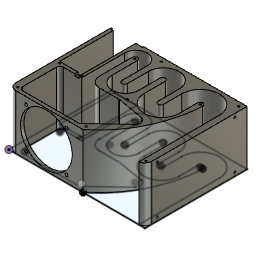
hifi_Back_horn_2_v2 v2 (Autodesk Fusion 360 design; units mm, degrees)
Autodesk Fusion 360 part; units mm, degrees
other "Fonction de maillage de base1"
sketch "Sketch1" plane through (0, 0, 0) normal (0, 0, 1) x (1, 0, 0)
  line L0 (0, 0) -> (200, 0)
  line L1 (200, 0) -> (200, 150)
  line L2 (200, 150) -> (0, 150)
  line L3 (0, 150) -> (0, 0)
  line L4 (42, 65) -> (42, 128)
  line L5 (53, 128) -> (53, 80)
  line L6 (61, 128) -> (61, 91)
  line L7 (75, 128) -> (75, 91)
  line L8 (83, 122) -> (83, 91)
  line L9 (100, 122) -> (100, 91)
  line L10 (108, 122) -> (108, 91)
  line L11 (128, 122) -> (128, 91)
  line L12 (136, 118) -> (136, 91)
  line L13 (159, 118) -> (159, 91)
  line L14 (191, 118) -> (191, 0)
  line L15 (136.3, 58.3) -> (97.4773, 65.0059)
  line L16 (140.5, 44.6) -> (99.9689, 6.2717)
  line L17 (96.6373, 5) -> (15, 5)
  line L18 (10, 10) -> (10, 60)
  line L19 (15, 65) -> (42, 65)
  line L20 (68, 65) -> (96.5085, 65)
  arc A0 (15, 65) -> (10, 60) centre (15, 60) ccw
  arc A1 (10, 10) -> (15, 5) centre (15, 10) ccw
  arc A2 (96.6373, 5) -> (99.9689, 6.2717) centre (96.6373, 10) ccw
  arc A3 (140.5, 44.6) -> (136.3, 58.3) centre (134.9332, 50.3872) ccw
  arc A4 (53, 80) -> (68, 65) centre (68, 80) ccw
  arc A5 (75, 91) -> (83, 91) centre (79, 91) ccw
  arc A6 (61, 91) -> (100, 91) centre (80.5, 91) ccw
  arc A7 (128, 122) -> (83, 122) centre (105.5, 122) ccw
  arc A8 (128, 91) -> (136, 91) centre (132, 91) ccw
  arc A9 (108, 91) -> (159, 91) centre (133.5, 91) ccw
  arc A10 (108, 122) -> (100, 122) centre (104, 122) ccw
  arc A11 (75, 128) -> (42, 128) centre (58.5, 128) ccw
  arc A12 (61, 128) -> (53, 128) centre (57, 128) ccw
  arc A13 (191, 118) -> (136, 118) centre (163.5, 118) ccw
  line L21 (96.5085, 65) -> (97.4773, 65.0059)
  spline S0 degree 5 poles (167, 118) (167, 115.0317) (166.6746, 108.5042) (165.211, 96.9417) (161.2879, 78.5371) (152.1463, 52.6808) (139.7381, 31.2801) (126.2481, 15.4712) (115.1076, 5.1248) (109, 0) knots 0 0 0 0 0 0 0.2 0.4 0.6 0.8 1 1 1 1 1 1
  line L22 (123.9379, 12.5344) -> (94.0621, -12.5344)
  line L23 (167, 125.2) -> (167, 110.8)
  arc A14 (167, 118) -> (159, 118) centre (163, 118) ccw
  line L24 (5, 150) -> (38, 150)
  line L25 (38, 150) -> (38, 69.5)
  line L26 (38, 69.5) -> (5, 69.5)
  line L27 (5, 69.5) -> (5, 150)
  line L28 (38, 69.5) -> (35, 69.5)
  line L29 (35, 69.5) -> (35, 65)
  line L30 (35, 65) -> (38, 65)
  line L31 (38, 65) -> (38, 69.5)
  point P0 (167, 118)
  dimension "d1" = 200
  dimension "d2" = 150
  dimension "d3" = 10
  dimension "d4" = 5
  dimension "d5" = 60
  dimension "d6" = 60
  dimension "d7" = 9
  dimension "d8" = 42
  dimension "d9" = 11
  dimension "d10" = 8
  dimension "d11" = 14
  dimension "d12" = 8
  dimension "d13" = 17
  dimension "d14" = 8
  dimension "d15" = 20
  dimension "d16" = 8
  dimension "d17" = 23
  dimension "d18" = 8
  dimension "d19" = 28
  dimension "d20" = 31
  dimension "d21" = 44.6
  dimension "d22" = 59.5
  dimension "d23" = 46.6
  dimension "d24" = 58.3
  dimension "d25" = 63.7
  dimension "d26" = 9.8
  dimension "d27" = 63
  dimension "d28" = 27
  dimension "d29" = 48
  dimension "d30" = 15
  dimension "d31" = 5
  dimension "d32" = 5
  dimension "d33" = 5
  dimension "d34" = 91
  dimension "d35" = 140
  dimension "d36" = 39
  dimension "d37" = 14.4
  dimension "d54" = 5
  dimension "d55" = 33
  dimension "d56" = 4.5
  dimension "d57" = 3
  constraint horizontal L0
  constraint vertical L1
  constraint horizontal L2
  constraint vertical L3
  constraint coincident L0.start L3.end
  constraint vertical L4
  constraint vertical L5
  constraint vertical L6
  constraint vertical L7
  constraint vertical L8
  constraint vertical L9
  constraint vertical L10
  constraint vertical L11
  constraint vertical L12
  constraint vertical L13
  constraint coincident L0 L14.end
  constraint perpendicular L0 L14
  constraint parallel L0 L17
  constraint perpendicular L17 L18
  constraint horizontal L20
  constraint horizontal L19
  constraint horizontal L13.start P0
  constraint horizontal L8.start L9.start
  constraint horizontal L9.start L10.start
  constraint horizontal L10.start L11.start
  constraint horizontal L7.end L8.end
  constraint horizontal L6.end L8.end
  constraint horizontal L6.end L10.end
  constraint horizontal L10.end L11.end
  constraint horizontal L11.end L12.end
  constraint horizontal L12.end L13.end
  constraint horizontal L8.end L9.end
  constraint tangent L18 A0
  constraint tangent L18 A1
  constraint tangent L17 A2
  constraint tangent L15 A3
  constraint tangent L20 A4
  constraint tangent L7 A5
  constraint tangent L6 A6
  constraint tangent L8 A7
  constraint tangent L11 A8
  constraint tangent L10 A9
  constraint tangent L9 A10
  constraint horizontal L5.start L6.start
  constraint horizontal L6.start L7.start
  constraint horizontal L4.end L5.start
  constraint tangent L4 A11
  constraint tangent L5 A12
  constraint horizontal L12.start L13.start
  constraint horizontal L14.start P0
  constraint tangent L12 A13
  constraint tangent L17 A1
  constraint tangent L19 A0
  constraint coincident P0 S0.start
  constraint coincident L0 S0.end
  constraint midpoint S0.end L22
  constraint midpoint P0 L23
  constraint vertical L23
  constraint tangent L13 A14
  constraint horizontal L24
  constraint vertical L25
  constraint horizontal L26
  constraint vertical L27
  constraint coincident L2 L24.start
  constraint horizontal L28
  constraint vertical L29
  constraint horizontal L30
  constraint vertical L31
  constraint coincident L19 L29.end
  measures "d1" distance of L0.start L0.end
  measures "d2" distance of L0.start L2.end
  measures "d3" distance of L3 L18
  measures "d4" distance of L0 L17
  measures "d5" distance of L17 L19
  measures "d6" distance of L17 L20
  measures "d7" distance of L1 L14
  measures "d8" distance of L3 L4
  measures "d9" distance of L4 L5
  measures "d10" distance of L5 L6
  measures "d11" distance of L6 L7
  measures "d12" distance of L7 L8
  measures "d13" distance of L8 L9
  measures "d14" distance of L9 L10
  measures "d15" distance of L10 L11
  measures "d16" distance of L11 L12
  measures "d17" distance of L12 L13
  measures "d18" distance of L13.start P0
  measures "d19" distance of L2 L9.start
  measures "d20" distance of L9.start L9.end
  measures "d21" distance of L0 L16.start
  measures "d22" distance of L1 L16.start
  measures "d23" angle of L1 L16
  measures "d24" distance of L0 L15.start
  measures "d25" distance of L1 L15.start
  measures "d26" angle of L15 L20
  measures "d27" distance of L4.start L4.end
  measures "d28" distance of L12.start L12.end
  measures "d29" distance of L5.start L5.end
  measures "d30" distance of L5 L20.start
  measures "d31" distance of L17 L18.start
  measures "d32" radius of A0
  measures "d33" radius of A2
  measures "d34" distance of L0.end S0.end
  measures "d35" angle of L0 L22
  measures "d36" distance of L22.start L22.end
  measures "d37" distance of L23.start L23.end
  measures "d54" distance of L3 L27
  measures "d55" distance of L25.end L26.end
  measures "d56" distance of L19 L26
  measures "d57" distance of L29 L31
extrude "Extrude1" add sketch "Sketch1" along normal blind 80 contours L0 L2 L3 L5 L6 L9 L10 L13 L15 L16 L17 L18 L19 L20 A0 A1 A2 A3 A4 A6 A9 A10 A12 L21 S0 A14 L26 L27 L29 | L0 L1 L2 L4 L7 L8 L11 L12 L14 L19 A5 A7 A8 A11 A13 L25 L31 | L19 L26 L28 L29 L30 L31
sketch "Sketch2" plane through (0, 0, 0) normal (0, 1, 0) x (1, 0, 0)
  circle A0 centre (55, -40) radius 38
  line L0 (42, 0) -> (75, 0)
  line L1 (55, -40) -> (55, 0) construction
  circle A1 centre (25.3015, -10.3015) radius 2.15
  line L2 (25.3015, -10.3015) -> (55, -40) construction
  circle A2 centre (25.3015, -69.6985) radius 2.15
  circle A3 centre (84.6985, -69.6985) radius 2.15
  circle A4 centre (84.6985, -10.3015) radius 2.15
  dimension "d40" = 76
  dimension "d41" = 40
  dimension "d42" = 55
  dimension "d43" = 4.3
  dimension "d44" = 42
  dimension "d45" = 45
  dimension "d47" = 360
  constraint coincident A0.centre L1.start
  constraint coincident L0 L1.end
  constraint vertical L1
  constraint coincident A1.centre L2.start
  measures "d40" diameter of A0
  measures "d41" distance of A0.centre L1.end
  measures "d42" distance of origin L1
  measures "d43" diameter of A1
  measures "d44" distance of A0.centre A1.centre
  measures "d45" angle of L1 L2
extrude "Extrude2" cut sketch "Sketch2" along normal up to surface (5 mm away)
fillet "Fillet1" radius 10 1 edges at (200, 0, 40)
fillet "Fillet2" radius 10 1 edges at (0, 0, 40)
extrude "Extrude3" cut sketch "Sketch1" against normal blind 3 from surface at 80 contours L19 L26 L28 L29 L30 L31
sketch "Sketch3" plane through (200, 0, 0) normal (1, 0, 0) x (0, 1, 0)
  line L0 (9.9499, 80) -> (9.9499, 0)
  line L1 (9.9499, 0) -> (150, 0)
  line L2 (150, 0) -> (150, 80)
  line L3 (150, 80) -> (9.9499, 80)
  circle A0 centre (18, 75) radius 1.5
  circle A1 centre (18, 5) radius 1.5
  circle A2 centre (132, 5) radius 1.5
  circle A3 centre (132, 75) radius 1.5
  line L4 (0, 0) -> (150, 0)
  line L5 (0, 0) -> (0, 80)
  dimension "d61" = 3
  dimension "d62" = 3
  dimension "d63" = 3
  dimension "d64" = 3
  dimension "d65" = 5
  dimension "d66" = 5
  dimension "d67" = 18
  dimension "d68" = 114
  constraint horizontal A1.centre A2.centre
  constraint horizontal A0.centre A3.centre
  constraint vertical A0.centre A1.centre
  constraint vertical A2.centre A3.centre
  measures "d61" diameter of A0
  measures "d62" diameter of A3
  measures "d63" diameter of A1
  measures "d64" diameter of A2
  measures "d65" distance of L3 A0.centre
  measures "d66" distance of A1.centre L4
  measures "d67" distance of A0.centre L5
  measures "d68" distance of A0.centre A3.centre
extrude "Extrude4" cut sketch "Sketch3" against normal blind 7 contours A0 | A1 | A2 | A3
sketch "Esquisse4" plane through (0, 65, 0) normal (0, -1, 0) x (1, 0, 0)
  line L0 (38, 80) -> (38, 77)
  line L1 (38, 77) -> (35, 77)
  line L2 (35, 77) -> (35, 80)
  line L3 (35, 80) -> (15, 80)
  line L4 (15, 80) -> (15, 0)
  line L5 (15, 0) -> (42, 0)
  line L6 (42, 0) -> (42, 80)
  line L7 (42, 80) -> (38, 80)
  line L8 (35, 80) -> (32, 80)
  line L9 (32, 80) -> (32, 77)
  line L10 (32, 77) -> (35, 77)
  line L11 (35, 77) -> (35, 80)
  constraint horizontal L8
  constraint vertical L9
  constraint horizontal L10
  constraint vertical L11
  constraint coincident L2.end L3.start
extrude "Extrusion5" cut sketch "Esquisse4" against normal blind 6 contours L2 L3 L8 L9 L10 L11
sketch "Esquisse5" plane through (0, 0, 80) normal (0, 0, 1) x (-1, 0, 0)
  line L0 (-32, -65) -> (-32, -69.5)
  line L1 (-32, -69.5) -> (-5, -69.5)
  line L2 (-5, -69.5) -> (-5, -150)
  line L3 (-5, -150) -> (0, -150)
  line L4 (0, -150) -> (0, -10)
  arc A0 (0, -10) -> (-10, 0) centre (-10, -10) ccw
  line L5 (-10, 0) -> (-109, 0)
  spline S0 degree 5 poles (-109, 0) (-115.1076, -5.1248) (-126.2481, -15.4712) (-139.7381, -31.2801) (-152.1463, -52.6808) (-161.2879, -78.5371) (-165.211, -96.9417) (-166.6746, -108.5042) (-167, -115.0317) (-167, -118) knots -1 -1 -1 -1 -1 -1 -0.8 -0.6 -0.4 -0.2 0 0 0 0 0 0
  arc A1 (-167, -118) -> (-159, -118) centre (-163, -118) ccw
  line L6 (-159, -118) -> (-159, -91)
  arc A2 (-108, -91) -> (-159, -91) centre (-133.5, -91) ccw
  line L7 (-108, -91) -> (-108, -122)
  arc A3 (-108, -122) -> (-100, -122) centre (-104, -122) ccw
  line L8 (-100, -122) -> (-100, -91)
  arc A4 (-61, -91) -> (-100, -91) centre (-80.5, -91) ccw
  line L9 (-61, -91) -> (-61, -128)
  arc A5 (-61, -128) -> (-53, -128) centre (-57, -128) ccw
  line L10 (-53, -128) -> (-53, -80)
  arc A6 (-53, -80) -> (-68, -65) centre (-68, -80) ccw
  line L11 (-68, -65) -> (-96.5085, -65)
  line L12 (-96.5085, -65) -> (-97.4773, -65.0059)
  line L13 (-97.4773, -65.0059) -> (-136.3, -58.3)
  arc A7 (-140.5, -44.6) -> (-136.3, -58.3) centre (-134.9332, -50.3872) ccw
  line L14 (-140.5, -44.6) -> (-99.9689, -6.2717)
  arc A8 (-96.6373, -5) -> (-99.9689, -6.2717) centre (-96.6373, -10) ccw
  line L15 (-96.6373, -5) -> (-15, -5)
  arc A9 (-10, -10) -> (-15, -5) centre (-15, -10) ccw
  line L16 (-10, -10) -> (-10, -60)
  arc A10 (-15, -65) -> (-10, -60) centre (-15, -60) ccw
  line L17 (-15, -65) -> (-32, -65)
  circle A11 centre (-7, -6) radius 1.35
  line L18 (0, -150) -> (0, 0)
  line L19 (0, 0) -> (-200, 0)
  circle A12 centre (-7, -67) radius 1.35
  line L20 (-38, -69.5) -> (-5, -69.5)
  circle A13 centre (-40.0341, -67) radius 1.35
  line L21 (-156.6564, -67) -> (-7, -67) construction
  circle A14 centre (-103.0854, -71) radius 1.35
  circle A15 centre (-57, -128) radius 1.35
  circle A16 centre (-163, -118) radius 1.35
  circle A17 centre (-107.3733, -6) radius 1.35
  circle A18 centre (-195.316, -6) radius 1.35
  circle A19 centre (-194, -144) radius 1.35
  circle A20 centre (-80, -144) radius 1.35
  line L22 (-200, -150) -> (0, -150)
  line L23 (-200, 0) -> (-200, -150)
  dimension "d73" = 2.7
  dimension "d74" = 7
  dimension "d75" = 6
  dimension "d76" = 2.7
  dimension "d77" = 7
  dimension "d78" = 2.5
  dimension "d79" = 2.7
  dimension "d81" = 2.7
  dimension "d83" = 4
  dimension "d86" = 2.7
  dimension "d87" = 2.7
  dimension "d88" = 2.7
  dimension "d89" = 6
  dimension "d90" = 2.7
  dimension "d91" = 6
  dimension "d92" = 2.7
  dimension "d93" = 2.7
  dimension "d94" = 6
  dimension "d95" = 6
  dimension "d96" = 6
  constraint coincident A12.centre L21.end
  constraint parallel L20 L21
  constraint coincident S0 L21.start
  constraint concentric A5 A15
  constraint concentric A1 A16
  measures "d73" diameter of A11
  measures "d74" distance of A11.centre L18
  measures "d75" distance of A11.centre L19
  measures "d76" diameter of A12
  measures "d77" distance of L18 A12.centre
  measures "d78" distance of A12.centre L20
  measures "d79" diameter of A13
  measures "d81" diameter of A14
  measures "d83" distance of L21 A14.centre
  measures "d86" diameter of A15
  measures "d87" diameter of A16
  measures "d88" diameter of A17
  measures "d89" distance of L19 A17.centre
  measures "d90" diameter of A18
  measures "d91" distance of L19 A18.centre
  measures "d92" diameter of A19
  measures "d93" diameter of A20
  measures "d94" distance of A20.centre L22
  measures "d95" distance of A19.centre L22
  measures "d96" distance of A19.centre L23
extrude "Extrusion6" cut sketch "Esquisse5" against normal blind 80 contours A11 | A12 | A13 | A14 | A15 | A16 | A17 | A18 | A19 | A20
sketch "Esquisse7" plane through (0, 150, 0) normal (0, 1, 0) x (-1, 0, 0)
  line L0 (-200, 0) -> (-38, 0)
  line L1 (-38, 0) -> (-38, 80)
  line L2 (-38, 80) -> (-200, 80)
  line L3 (-200, 80) -> (-200, 0)
  line L4 (-38, 80) -> (-48, 80)
  line L5 (-48, 80) -> (-48, 0)
  line L6 (-48, 0) -> (-38, 0)
  line L7 (-38, 0) -> (-38, 80)
  line L8 (-5, 80) -> (-2, 80)
  line L9 (-2, 80) -> (-2, -0.2021)
  line L10 (-2, -0.2021) -> (-5, -0.2021)
  line L11 (-5, -0.2021) -> (-5, 80)
  dimension "d99" = 10
  dimension "d102" = 3
  constraint horizontal L4
  constraint vertical L5
  constraint horizontal L6
  constraint vertical L7
  constraint coincident L1.end L2.start
  constraint horizontal L8
  constraint vertical L9
  constraint horizontal L10
  constraint vertical L11
  measures "d99" distance of L1.end L4.end
  measures "d102" distance of L8.start L8.end
extrude "Extrusion7" cut sketch "Esquisse7" against normal blind 1.5 contours L0 L1 L2 L4 L5 L6 L7
extrude "Extrusion8" cut sketch "Esquisse7" against normal blind 1.5 contours L8 L9 L10 L11
sketch "Esquisse8" plane through (43, 150, 40) normal (0, 1, 0) x (-1, 0, 0)
  circle A0 centre (0, 30) radius 1.35
  line L0 (5, -40) -> (5, 40)
  line L1 (5, 40) -> (-5, 40)
  line L2 (-5, 0) -> (5, 0) construction
  circle A1 centre (0, -30) radius 1.35
  dimension "d105" = 2.7
  dimension "d106" = 5
  dimension "d107" = 10
  constraint midpoint L0 L2.end
  constraint perpendicular L0 L2
  constraint symmetric A0 L2 A1
  measures "d105" diameter of A0
  measures "d106" distance of A0.centre L0
  measures "d107" distance of A0.centre L1
extrude "Extrusion9" cut sketch "Esquisse8" against normal blind 10
equation "d76 = d73"
equation "d77 = d74"
equation "d79 = d73"
equation "d81 = d73"
equation "d86 = d73"
equation "d87 = d73"
equation "d88 = d73"
equation "d89 = d75"
equation "d90 = d73"
equation "d91 = d89"
equation "d92 = d73"
equation "d93 = d73"
equation "d94 = d75"
equation "d95 = d75"
equation "d96 = d75"
equation "d105 = d73"
